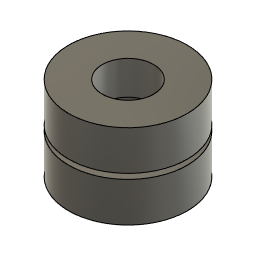
Numisheet_BM-1 (Autodesk Fusion 360 design; units mm, degrees)
Autodesk Fusion 360 part; units mm, degrees
sketch "Sketch1" plane through (0, 0, 0) normal (0, 0, 1) x (1, 0, 0) in component "Blank"
  line L0 (15, 0) -> (107.5, 0)
  line L1 (107.5, 0) -> (107.5, 1.2)
  line L2 (107.5, 1.2) -> (15, 1.2)
  line L3 (15, 1.2) -> (15, 0)
  line L4 (0, 0) -> (15, 0) construction
  dimension "d1" = 15
  dimension "d2" = 1.2
  dimension "d3" = 107.5
  constraint coincident L4.start origin
  constraint horizontal L0
  constraint vertical L1
  constraint horizontal L2
  constraint vertical L3
  constraint perpendicular L3 L4
  measures "d1" distance of L3 L4.start
  measures "d2" distance of L0.end L1.end
  measures "d3" distance of L4.start L0.end
sketch "Sketch1 (2)" plane through (0, 0, 0) normal (0, 0, 1) x (1, 0, 0) in component "Punch"
  line L0 (0, -1) -> (35, -1)
  arc A0 (50, -16) -> (35, -1) centre (35, -16) ccw
  line L1 (50, -16) -> (50, -101)
  line L2 (50, -101) -> (0, -101)
  line L3 (0, -101) -> (0, -1)
  line L4 (0, 0) -> (0, -1) construction
  dimension "d4" = 1
  dimension "d5" = 15
  dimension "d6" = 50
  dimension "d7" = 100
  constraint horizontal L0
  constraint tangent L0 A0
  constraint perpendicular L0 L1
  constraint perpendicular L1 L2
  constraint perpendicular L0 L3
  constraint coincident L4.start origin
  constraint perpendicular L0 L4
  constraint tangent A0 L1
  measures "d4" distance of L0.start L4.start
  measures "d5" radius of A0
  measures "d6" distance of L1 L3
  measures "d7" distance of L0 L2
revolve "Revolve1" add sketch "Sketch1" angle 360 about axis through (0, 1.75, 0) along (0, 1, 0) makes body 1 in component "Blank"
revolve "Revolve1'" add sketch "Sketch1 (2)" angle 360 about axis through (0, 1.75, 0) along (0, 1, 0) separate body makes body 2 in component "Punch"
sketch "Sketch1 (3)" plane through (0, 0, 0) normal (0, 0, 1) x (1, 0, 0) in component "Lower Die"
  line L0 (150, -101) -> (51, -101)
  line L1 (51, -101) -> (51, -1)
  line L2 (150, -1) -> (150, -101)
  line L3 (0, 0) -> (145.9658, 0) construction
  line L4 (95, -3) -> (95, -7)
  line L5 (95, -7) -> (100, -7)
  line L6 (100, -7) -> (100, -3)
  line L7 (51, -1) -> (93, -1)
  line L8 (102, -1) -> (150, -1)
  arc A0 (95, -3) -> (93, -1) centre (93, -3) ccw
  arc A1 (102, -1) -> (100, -3) centre (102, -3) ccw
  line L9 (0, 0) -> (0, -124.5009) construction
  dimension "d10" = 1
  dimension "d11" = 100
  dimension "d12" = 5
  dimension "d13" = 6
  dimension "d14" = 2
  dimension "d15" = 95
  dimension "d16" = 51
  dimension "d17" = 150
  constraint horizontal L0
  constraint vertical L1
  constraint horizontal L7
  constraint vertical L2
  constraint coincident L3.start L9.start
  constraint parallel L3 L7
  constraint perpendicular L4 L7
  constraint perpendicular L4 L5
  constraint perpendicular L6 L7
  constraint collinear L7 L8
  constraint tangent L4 A0
  constraint tangent L7 A0
  constraint tangent L6 A1
  constraint tangent L8 A1
  constraint equal A0 A1
  constraint perpendicular L3 L9
  measures "d10" distance of L3 L7
  measures "d11" distance of L0.start L2.start
  measures "d12" distance of L4.end L5.end
  measures "d13" distance of L5 L8
  measures "d14" radius of A0
  measures "d15" distance of L4 L9
  measures "d16" distance of L1 L9
  measures "d17" distance of L2 L9
revolve "Revolve1''" add sketch "Sketch1 (3)" angle 360 about axis through (0, 1.75, 0) along (0, 1, 0) separate body makes body 3 in component "Lower Die"
sketch "Sketch1 (4)" plane through (0, 0, 0) normal (0, 0, 1) x (1, 0, 0) in component "Upper Die"
  line L0 (130, 0) -> (0, 0) construction
  line L1 (0, 0) -> (0, 125) construction
  line L2 (65, 27.2) -> (65, 112.2)
  line L3 (65, 112.2) -> (150, 112.2)
  line L4 (150, 112.2) -> (150, 12.2)
  arc A0 (65, 27.2) -> (80, 12.2) centre (80, 27.2) ccw
  line L5 (103.7642, 12.2) -> (106.1888, 12.2)
  line L6 (95.5774, 11.2) -> (96.634, 9.3699)
  line L7 (98.366, 9.3699) -> (99.4226, 11.2)
  line L8 (150, 12.2) -> (101.1547, 12.2)
  line L9 (93.8453, 12.2) -> (80, 12.2)
  arc A1 (95.5774, 11.2) -> (93.8453, 12.2) centre (93.8453, 10.2) ccw
  arc A2 (101.1547, 12.2) -> (99.4226, 11.2) centre (101.1547, 10.2) ccw
  arc A3 (96.634, 9.3699) -> (98.366, 9.3699) centre (97.5, 9.8699) ccw
  line L10 (101.1547, 12.2) -> (93.8453, 12.2) construction
  line L11 (95.5774, 11.2) -> (95, 12.2) construction
  line L12 (99.4226, 11.2) -> (100, 12.2) construction
  point P0 (100, 12.2)
  point P1 (95, 12.2)
  dimension "d19" = 12.2
  dimension "d20" = 15
  dimension "d21" = 100
  dimension "d22" = 65
  dimension "d23" = 60
  dimension "d24" = 120
  dimension "d25" = 2
  dimension "d27" = 1
  dimension "d28" = 95
  dimension "d29" = 100
  dimension "d30" = 150
  constraint coincident L0.end L1.start
  constraint horizontal L0
  constraint perpendicular L0 L1
  constraint horizontal L8
  constraint vertical L2
  constraint horizontal L3
  constraint vertical L4
  constraint tangent A0 L8
  constraint tangent L2 A0
  constraint coincident L5.start L8
  constraint coincident L5.end L8
  constraint collinear L8 L9
  constraint tangent L9 A1
  constraint tangent L6 A1
  constraint tangent L8 A2
  constraint tangent L7 A2
  constraint tangent L6 A3
  constraint tangent L7 A3
  constraint equal A1 A2
  constraint coincident L10 P1
  constraint coincident L10 P0
  constraint parallel L6 L11
  constraint parallel L7 L12
  constraint coincident L11 P1
  constraint coincident L12 P0
  measures "d19" distance of L0 L8
  measures "d20" radius of A0
  measures "d21" distance of L4.end L3.end
  measures "d22" distance of L1 L2
  measures "d23" angle of L6 L7
  measures "d24" angle of L6 L9
  measures "d25" radius of A1
  measures "d27" radius of A3
  measures "d28" distance of L1 P1
  measures "d29" distance of L1 P0
  measures "d30" distance of L1 L4
revolve "Revolve1'''" add sketch "Sketch1 (4)" angle 360 about axis through (0, 0, 0) along (0, 1, 0) separate body makes body 4 in component "Upper Die"
component "Blank" placed x (1, 0, 0) y (0, 1, 0) z (0, 0, 1) at (0, 0, 0)
component "Punch" placed x (1, 0, 0) y (0, 1, 0) z (0, 0, 1) at (0, 0, 0)
component "Lower Die" placed x (1, 0, 0) y (0, 1, 0) z (0, 0, 1) at (0, 0, 0)
component "Upper Die" placed x (1, 0, 0) y (0, 1, 0) z (0, 0, 1) at (0, 0, 0)
